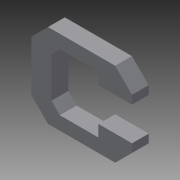
# Autodesk Inventor part: HW 4 Part 1
Saved by Autodesk Inventor 2015 SP1 (Build 190203100, 203)
## iProperties
Created: 2016-01-25
Part Number: HW 4 Part 1
Material: Generic
Document SubType Name: Modeling
Designer: melissa.roth
Density: 1 g/cm^3
Appearance: Default
Author: melissa.roth
Autodesk Inventor part; units mm, degrees
ref_plane "YZ Plane" through (0, 0, 0) normal (1, 0, 0) x (0, 1, 0)
ref_plane "XZ Plane" through (0, 0, 0) normal (0, 1, 0) x (-1, 0, 0)
ref_plane "XY Plane" through (0, 0, 0) normal (0, 0, 1) x (1, 0, 0)
sketch "Sketch1" plane through (0, 0, 0) normal (0, 0, 1) x (1, 0, 0)
  line L0 (0, 0) -> (25.4, 0)
  line L1 (25.4, 0) -> (31.75, 6.35)
  line L2 (31.75, 6.35) -> (31.75, 9.525)
  line L3 (31.75, 9.525) -> (19.05, 9.525)
  line L4 (19.05, 9.525) -> (19.05, 5.08)
  line L5 (19.05, 5.08) -> (4.445, 5.08)
  line L6 (4.445, 5.08) -> (1.27, 8.255)
  line L7 (1.27, 8.255) -> (1.27, 23.495)
  line L8 (1.27, 23.495) -> (4.445, 26.67)
  line L9 (4.445, 26.67) -> (19.05, 26.67)
  line L10 (19.05, 26.67) -> (19.05, 22.225)
  line L11 (19.05, 22.225) -> (31.75, 22.225)
  line L12 (31.75, 22.225) -> (31.75, 25.4)
  line L13 (31.75, 25.4) -> (25.4, 31.75)
  line L14 (25.4, 31.75) -> (0, 31.75)
  line L15 (0, 31.75) -> (-6.35, 25.4)
  line L16 (-6.35, 25.4) -> (-6.35, 6.35)
  line L17 (-6.35, 6.35) -> (0, 0)
  dimension "d0" = 31.75
  dimension "d1" = 31.75
  dimension "d2" = 45
  dimension "d3" = 45
  dimension "d4" = 31.75
  dimension "d5" = 38.1
  dimension "d6" = 38.1
  dimension "d8" = 9.525
  dimension "d9" = 9.525
  dimension "d10" = 12.7
  dimension "d11" = 5.08
  dimension "d12" = 5.08
  dimension "d13" = 3.175
  dimension "d14" = 3.175
  dimension "d15" = 45
  dimension "d16" = 45
  dimension "d17" = 12.7
  dimension "d18" = 6.35
  dimension "d19" = 6.35
  dimension "d20" = 7.62
  constraints: 36 end point, 4 parallel, 3 point on line, 2 equal length, 2 perpendicular, 1 horizontal
  measures "d0" horizontal distance of L13.end L15.end
  measures "d1" horizontal distance of L0.end L16.end
  measures "d2" angle of L13 L14
  measures "d3" angle of L1 L0
  measures "d4" distance of L0.start L14.end
  measures "d5" distance of L1.end L16.end
  measures "d6" distance of L12.end L15.end
  measures "d8" vertical distance of L0.end L2.end
  measures "d9" vertical distance of L13.end L11.end
  measures "d10" distance between parallel lines of L3 L11
  measures "d11" distance between parallel lines of L0 L5
  measures "d12" distance between parallel lines of L14 L9
  measures "d13" horizontal distance of L8.end L7.end
  measures "d14" horizontal distance of L5.end L6.end
  measures "d15" angle of L8 L7
  measures "d16" angle of L6 L7
  measures "d17" distance of L2.end L3.end
  measures "d18" horizontal distance of L14.end L15.end
  measures "d19" horizontal distance of L14.end L15.end
  measures "d20" distance between parallel lines of L7 L16
extrude "Extrusion1" add sketch "Sketch1" along normal blind 6.35
body "Solid1"
